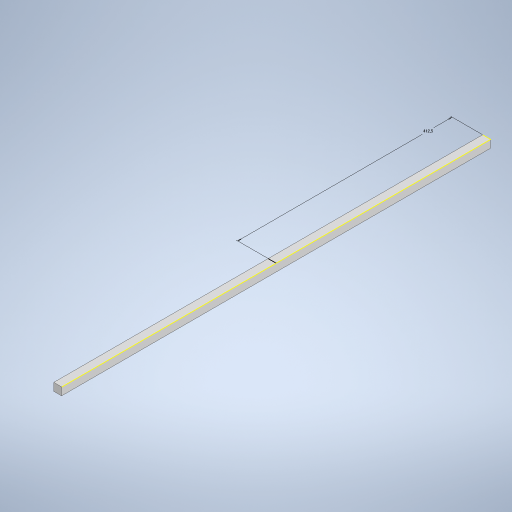
# Autodesk Inventor part: 試作_825
Saved by Autodesk Inventor 2023 (Build 270158000, 158)
## iProperties
Created: 2022-04-26
Part Number: 試作_825
Material: 一般
Document SubType Name: Modeling
Designer: yuta
Density: 1 g/cm^3
Appearance: 既定
Mass: 185.625 g
Surface Area: 499.5 cm^2
Volume: 185.625 cm^3
Author: yuta
Autodesk Inventor part; units mm, degrees
ref_plane "YZ Plane" through (0, 0, 0) normal (1, 0, 0) x (0, 1, 0)
ref_plane "XZ Plane" through (0, 0, 0) normal (0, 1, 0) x (-1, 0, 0)
ref_plane "XY Plane" through (0, 0, 0) normal (0, 0, 1) x (1, 0, 0)
sketch "スケッチ1" plane through (0, 0, 0) normal (0, 0, 1) x (1, 0, 0)
  line L0 (0, 0) -> (15, 0)
  line L1 (15, 0) -> (15, 15)
  line L2 (15, 15) -> (0, 15)
  line L3 (0, 15) -> (0, 0)
  dimension "d0" = 15
  dimension "d1" = 15
  constraints: 8 end point, 2 parallel, 1 horizontal, 1 perpendicular
  measures "d0" distance of L2.end L1.end
  measures "d1" distance of L1.end L0.end
extrude "押し出し1" add sketch "スケッチ1" along normal blind 825
sketch "スケッチ2" plane through (0, 15, 825) normal (0, 1, 0) x (1, 0, 0)
  line L0 (0, 412.5) -> (15, 412.5)
  line L1 (15, 825) -> (15, 0) projected
  line L2 (15, 825) -> (0, 825) projected
  dimension "d5" = 412.5
  constraints: 2 end point, 1 midpoint
  measures "d5" distance between parallel lines of L2 L0
